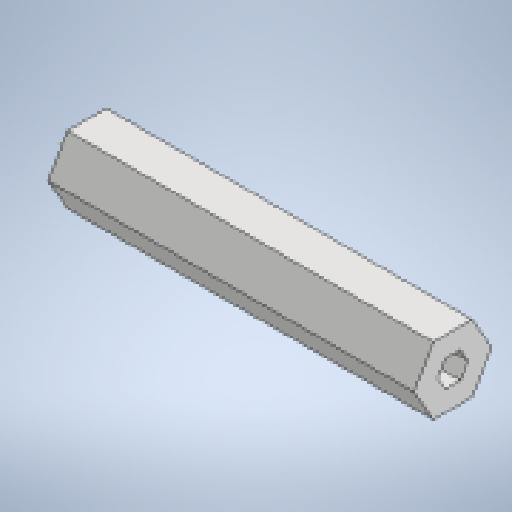
# Autodesk Inventor part: 500H x 50mm
Saved by Autodesk Inventor 2023 (Build 270158000, 158)
## iProperties
Created: 2021-10-04
Part Number: 500H x 50mm
Material: Generic
Document SubType Name: Modeling
Designer: TakeHomePC
Density: 1 g/cm^3
Appearance: Default
Author: TakeHomePC
Autodesk Inventor part; units mm, degrees
ref_plane "YZ Plane" through (0, 0, 0) normal (1, 0, 0) x (0, 1, 0)
ref_plane "XZ Plane" through (0, 0, 0) normal (0, 1, 0) x (-1, 0, 0)
ref_plane "XY Plane" through (0, 0, 0) normal (0, 0, 1) x (1, 0, 0)
sketch "Sketch1" plane through (0, 0, 0) normal (1, 0, 0) x (0, 1, 0)
  line L0 (-6.35, -3.6662) -> (0, -7.3323)
  line L1 (-6.35, 3.6662) -> (-6.35, -3.6662)
  line L2 (0, 7.3323) -> (-6.35, 3.6662)
  line L3 (6.35, 3.6662) -> (0, 7.3323)
  line L4 (6.35, -3.6662) -> (6.35, 3.6662)
  line L5 (0, -7.3323) -> (6.35, -3.6662)
  line L6 (2.5, -1.4434) -> (0, -2.8868)
  line L7 (0, -2.8868) -> (-2.5, -1.4434)
  line L8 (-2.5, -1.4434) -> (-2.5, 1.4434)
  line L9 (-2.5, 1.4434) -> (0, 2.8868)
  line L10 (0, 2.8868) -> (2.5, 1.4434)
  line L11 (2.5, 1.4434) -> (2.5, -1.4434)
  point P0 (0, 0)
  point P1 (0, 0)
  dimension "d0" = 5
  constraints: 24 end point, 1 coincident, 13 other
  measures "d0" distance between parallel lines of L8 L11
extrude "Extrusion1" add sketch "Sketch1" along normal blind 69.0855
body "Solid1"
